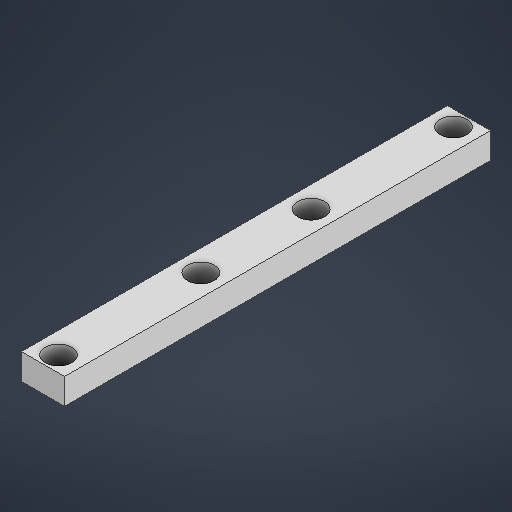
# Autodesk Inventor part: peça3
Saved by Autodesk Inventor 2026 (Build 300175000, 175)
## iProperties
Created: 2026-04-17
Part Number: peça3
Material: Genérico
Document SubType Name: Modeling
Designer: a2453266
Density: 1 g/cm^3
Appearance: Padrão
Author: a2453266
Autodesk Inventor part; units mm, degrees
ref_plane "YZ Plane" through (0, 0, 0) normal (1, 0, 0) x (0, 1, 0)
ref_plane "XZ Plane" through (0, 0, 0) normal (0, 1, 0) x (-1, 0, 0)
ref_plane "XY Plane" through (0, 0, 0) normal (0, 0, 1) x (1, 0, 0)
sketch "Esboço1" plane through (0, 0, 0) normal (0, 1, 0) x (-1, 0, 0)
  line L0 (0, 0) -> (5, 0)
  line L1 (5, 0) -> (5, -49.4)
  line L2 (5, -49.4) -> (0, -49.4)
  line L3 (0, -49.4) -> (0, 0)
  dimension "d0" = 5
  dimension "d1" = 49.4
  constraints: 8 end point, 2 parallel, 1 horizontal, 1 perpendicular
  measures "d0" distance of L1.end L2.end
  measures "d1" distance of L0.end L1.end
extrude "Extrusão1" add sketch "Esboço1" along normal blind 3
sketch "Esboço2" plane through (0, 3, 0) normal (0, 1, 0) x (1, 0, 0)
  line L0 (-5, 0) -> (0, 0) projected
  line L1 (-2.5, 0) -> (-2.5, 1.8)
  line L2 (0, 49.4) -> (-5, 49.4) projected
  line L3 (-2.5, 49.4) -> (-2.5, 47.6)
  circle A0 centre (-2.5, 1.8) radius 1.55
  circle A1 centre (-2.5, 47.6) radius 1.55
  line L4 (-5, 0) -> (-5, 18.3)
  line L5 (-5, 49.4) -> (-5, 0) projected
  line L6 (-5, 49.4) -> (-5, 31.1)
  line L7 (-5, 18.3) -> (0, 18.3)
  line L8 (-5, 31.1) -> (0, 31.1)
  line L9 (0, 0) -> (0, 49.4) projected
  circle A2 centre (-2.5, 18.3) radius 1.55
  circle A3 centre (-2.5, 31.1) radius 1.55
  dimension "d4" = 1.8
  dimension "d5" = 1.8
  dimension "d6" = 3.1
  dimension "d7" = 3.1
  dimension "d8" = 18.3
  dimension "d9" = 18.3
  dimension "d10" = 3.1
  dimension "d11" = 3.1
  constraints: 12 end point, 4 centre point, 4 midpoint, 3 point on line, 2 coincident, 2 horizontal, 2 vertical
  measures "d4" distance of L1.start L1.end
  measures "d5" distance of L3.start L3.end
  measures "d6" diameter of A0
  measures "d7" diameter of A1
  measures "d8" distance of L0.start L4.end
  measures "d9" distance of L2.end L6.end
  measures "d10" diameter of A2
  measures "d11" diameter of A3
extrude "Extrusão2" cut sketch "Esboço2" against normal blind 3 contours A0 | A1 | A2 L7 | L7 A2 | A3 L8 | L8 A3
